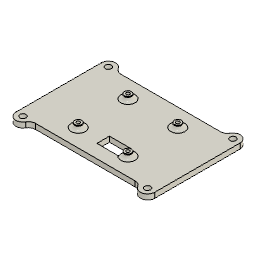
ELP Camera Mount Topside (Autodesk Fusion 360 design; units mm, degrees)
Autodesk Fusion 360 part; units mm, degrees
sketch "Sketch1" plane through (0, 0, 0) normal (0, 0, 1) x (1, 0, 0)
  line L0 (35, -24) -> (-35, -24) construction
  line L1 (-35, -24) -> (-35, 24) construction
  line L2 (-35, 24) -> (35, 24) construction
  line L3 (35, 24) -> (35, -24) construction
  line L4 (35, -24) -> (-35, 24) construction
  line L5 (-35, -24) -> (35, 24) construction
  line L6 (28, -28) -> (-28, -28) construction
  line L7 (-28, -28) -> (-28, 28) construction
  line L8 (-28, 28) -> (28, 28) construction
  line L9 (28, 28) -> (28, -28) construction
  line L10 (28, -28) -> (-28, 28) construction
  line L11 (-28, -28) -> (28, 28) construction
  circle A0 centre (-35, 24) radius 1.7
  circle A1 centre (35, 24) radius 1.7
  circle A2 centre (35, -24) radius 1.7
  circle A3 centre (-35, -24) radius 1.7
  circle A4 centre (-28, -28) radius 4
  circle A5 centre (-28, 28) radius 4
  circle A6 centre (28, 28) radius 4
  circle A7 centre (28, -28) radius 4
  circle A8 centre (35, -24) radius 4.0623
  circle A9 centre (-35, -24) radius 4.0623
  circle A10 centre (-35, 24) radius 4.0623
  circle A11 centre (35, 24) radius 4.0623
  line L12 (39.0623, 24) -> (39.0623, -24)
  line L13 (-39.0623, 24) -> (-39.0623, -24)
  line L14 (-28, 24) -> (28, 24)
  line L15 (-28, -24) -> (28, -24)
  dimension "d1" = 70
  dimension "d2" = 48
  dimension "d3" = 56
  dimension "d4" = 56
  dimension "d5" = 3.4
  dimension "d6" = 3.4
  dimension "d7" = 3.4
  dimension "d8" = 3.4
  dimension "d9" = 8
  dimension "d10" = 8
  dimension "d11" = 8
  dimension "d12" = 8
  constraint horizontal L0
  constraint perpendicular L0 L1
  constraint parallel L0 L2
  constraint parallel L1 L3
  constraint coincident L4 origin
  constraint coincident L5 origin
  constraint horizontal L6
  constraint perpendicular L6 L7
  constraint parallel L6 L8
  constraint parallel L7 L9
  constraint coincident L10 origin
  constraint coincident L11 origin
  constraint coincident L1.end L2.start
  constraint coincident L2.end L3.start
  constraint coincident L0.start L3.end
  constraint coincident L0.end L1.start
  constraint coincident L6.end L7.start
  constraint coincident L7.end L8.start
  constraint coincident L8.end L9.start
  constraint coincident L6.start L9.end
  constraint concentric A2 A8
  constraint tangent A7 A8
  constraint concentric A3 A9
  constraint tangent A4 A9
  constraint concentric A0 A10
  constraint tangent A5 A10
  constraint concentric A1 A11
  constraint tangent A6 A11
  constraint coincident A11 L12.start
  constraint coincident A8 L12.end
  constraint tangent A8 L12
  constraint tangent A11 L12
  constraint coincident A10 L13.start
  constraint coincident A9 L13.end
  constraint vertical L13
  constraint tangent A10 L13
  constraint coincident A5 L14.start
  constraint coincident L7 L14.start
  constraint coincident A6 L14.end
  constraint coincident L9 L14.end
  constraint coincident L7 L15.start
  constraint coincident L0 L15.start
  constraint coincident A7 L15.end
  constraint coincident L9 L15.end
  measures "d1" distance of L1.end L2.end
  measures "d2" distance of L0.end L1.end
  measures "d3" distance of L7.end L8.end
  measures "d4" distance of L6.end L7.end
  measures "d5" diameter of A0
  measures "d6" diameter of A1
  measures "d7" diameter of A2
  measures "d8" diameter of A3
  measures "d9" diameter of A4
  measures "d10" diameter of A5
  measures "d11" diameter of A6
  measures "d12" diameter of A7
extrude "Extrude1" add sketch "Sketch1" along normal blind 3 contours A4 A5 A6 A7 A8 A9 A10 A11 L12 L13 L14 L15 | A9 | A8 | A10 | A11
sketch "Sketch2" plane through (0, 0, 3) normal (0, 0, 1) x (-1, 0, 0)
  circle A0 centre (35, -24) radius 1.7
  circle A1 centre (35, 24) radius 1.7
  circle A2 centre (-35, -24) radius 1.7
  circle A3 centre (-35, 24) radius 1.7
  arc A4 (31.473, -26.0154) -> (39.0623, -24) centre (35, -24) ccw
  line L0 (39.0623, -24) -> (39.0623, 24)
  arc A5 (39.0623, 24) -> (31.473, 26.0154) centre (35, 24) ccw
  arc A6 (28, 24) -> (31.473, 26.0154) centre (28, 28) ccw
  line L1 (28, 24) -> (-28, 24)
  arc A7 (-31.473, 26.0154) -> (-28, 24) centre (-28, 28) ccw
  arc A8 (-31.473, 26.0154) -> (-39.0623, 24) centre (-35, 24) ccw
  line L2 (-39.0623, 24) -> (-39.0623, -24)
  arc A9 (-39.0623, -24) -> (-31.473, -26.0154) centre (-35, -24) ccw
  arc A10 (-28, -24) -> (-31.473, -26.0154) centre (-28, -28) ccw
  line L3 (-28, -24) -> (28, -24)
  arc A11 (31.473, -26.0154) -> (28, -24) centre (28, -28) ccw
  line L4 (-14, 14) -> (14, 14) construction
  line L5 (14, 14) -> (14, -14) construction
  line L6 (14, -14) -> (-14, -14) construction
  line L7 (-14, -14) -> (-14, 14) construction
  line L8 (-14, 14) -> (14, -14) construction
  line L9 (14, 14) -> (-14, -14) construction
  circle A12 centre (-14, -14) radius 0.95
  circle A13 centre (14, -14) radius 0.95
  circle A14 centre (14, 14) radius 0.95
  circle A15 centre (-14, 14) radius 0.95
  circle A16 centre (-14, -14) radius 2
  circle A17 centre (14, -14) radius 2
  circle A18 centre (14, 14) radius 2
  circle A19 centre (-14, 14) radius 2
  dimension "d15" = 28
  dimension "d16" = 28
  dimension "d17" = 1.9
  dimension "d18" = 1.9
  dimension "d19" = 1.9
  dimension "d20" = 1.9
  dimension "d21" = 4
  dimension "d22" = 4
  dimension "d23" = 4
  dimension "d24" = 4
  constraint horizontal L4
  constraint perpendicular L4 L5
  constraint parallel L4 L6
  constraint parallel L5 L7
  constraint coincident L8 origin
  constraint coincident L9 origin
  constraint coincident L6.end L7.start
  constraint coincident L5.end L6.start
  constraint coincident L4.end L5.start
  constraint coincident L4.start L7.end
  constraint concentric A12 A16
  constraint concentric A13 A17
  constraint concentric A14 A18
  constraint concentric A15 A19
  measures "d15" distance of L5.end L6.end
  measures "d16" distance of L4.end L5.end
  measures "d17" diameter of A12
  measures "d18" diameter of A13
  measures "d19" diameter of A14
  measures "d20" diameter of A15
  measures "d21" diameter of A16
  measures "d22" diameter of A17
  measures "d23" diameter of A18
  measures "d24" diameter of A19
extrude "Extrude2" cut sketch "Sketch2" against normal up to surface (3 mm away) contours A12 | A13 | A14 | A15
extrude "Extrude3" add sketch "Sketch2" along normal blind 2.5 contours A16 | A17 | A18 | A19
sketch "Sketch3" plane through (0, 0, 3) normal (0, 0, 1) x (-1, 0, 0)
  circle A0 centre (-14, 14) radius 2
  circle A1 centre (14, 14) radius 2
  circle A2 centre (-14, -14) radius 2
  circle A3 centre (14, -14) radius 2
  circle A4 centre (35, -24) radius 1.7
  circle A5 centre (35, 24) radius 1.7
  circle A6 centre (-35, -24) radius 1.7
  circle A7 centre (-35, 24) radius 1.7
  arc A8 (31.473, -26.0154) -> (39.0623, -24) centre (35, -24) ccw
  line L0 (39.0623, -24) -> (39.0623, 24)
  arc A9 (39.0623, 24) -> (31.473, 26.0154) centre (35, 24) ccw
  arc A10 (28, 24) -> (31.473, 26.0154) centre (28, 28) ccw
  line L1 (28, 24) -> (-28, 24)
  arc A11 (-31.473, 26.0154) -> (-28, 24) centre (-28, 28) ccw
  arc A12 (-31.473, 26.0154) -> (-39.0623, 24) centre (-35, 24) ccw
  line L2 (-39.0623, 24) -> (-39.0623, -24)
  arc A13 (-39.0623, -24) -> (-31.473, -26.0154) centre (-35, -24) ccw
  arc A14 (-28, -24) -> (-31.473, -26.0154) centre (-28, -28) ccw
  line L3 (-28, -24) -> (28, -24)
  arc A15 (31.473, -26.0154) -> (28, -24) centre (28, -28) ccw
  line L4 (0, -30) -> (0, 29.88) construction
  line L5 (45.0284, -0.06) -> (-45.0979, -0.06) construction
  line L6 (-11, 16.44) -> (1, 16.44)
  line L7 (1, 16.44) -> (1, 9.44)
  line L8 (1, 9.44) -> (-11, 9.44)
  line L9 (-11, 9.44) -> (-11, 16.44)
  line L10 (-11, 16.44) -> (1, 9.44) construction
  line L11 (1, 16.44) -> (-11, 9.44) construction
  point P0 (-5, 12.94)
  dimension "d29" = 12
  dimension "d30" = 7
  dimension "d31" = 13
  dimension "d32" = 5
  constraint perpendicular L1 L4
  constraint perpendicular L4 L5
  constraint horizontal L6
  constraint perpendicular L6 L7
  constraint parallel L6 L8
  constraint parallel L7 L9
  constraint coincident L10 P0
  constraint coincident L11 P0
  measures "d29" distance of L7.end L8.end
  measures "d30" distance of L6.end L7.end
  measures "d31" distance of L5 P0
  measures "d32" distance of L4 P0
extrude "Extrude4" cut sketch "Sketch3" against normal up to surface (3 mm away) contours L6 L7 L8 L9
fillet "Fillet1" radius 2 4 edges at (15.8647, -14.7232, 3) (15.8647, 13.2768, 3) (-12.1353, 13.2768, 3) (-12.1353, -14.7232, 3)
